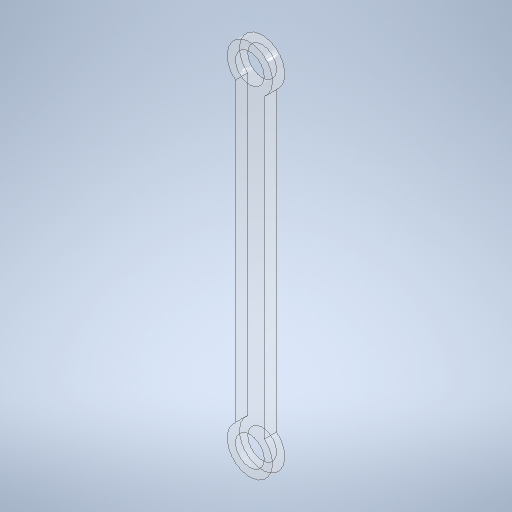
# Autodesk Inventor part: 4P.01.02.28-BC-v1-Final Aileron L3 80deg
Saved by Autodesk Inventor 2025.2 (Build 292293000, 293)
## iProperties
Created: 2025-01-30
Part Number: 4P.01.02.28-BC-v1-Final Aileron L3 80deg
Material: Acrylic, Clear
Document SubType Name: Modeling
Designer: Carriett 4
Density: 1.19 g/cm^3
Appearance: Transparent - Clear
Category: <PART CATAGORY>
Title: <TITLE>
Author: Carriett 4
Revision Number: 1
Autodesk Inventor part; units mm, degrees
ref_plane "YZ Plane" through (0, 0, 0) normal (1, 0, 0) x (0, 1, 0)
ref_plane "XZ Plane" through (0, 0, 0) normal (0, 1, 0) x (-1, 0, 0)
ref_plane "XY Plane" through (0, 0, 0) normal (0, 0, 1) x (1, 0, 0)
sketch "Sketch6" plane through (0, 0, 0) normal (0, 0, 1) x (1, 0, 0)
  arc A0 (9, 81.8659) -> (2, 81.8659) centre (5.5, 86.1086) ccw
  arc A1 (2, 9.7426) -> (9, 9.7426) centre (5.5, 5.5) ccw
  circle A2 centre (5.5, 5.5) radius 3.5
  circle A3 centre (5.5, 86.1086) radius 3.5
  line L0 (2, 81.8659) -> (2, 9.7426)
  line L1 (9, 9.7426) -> (9, 81.8659)
  point P0 (0, 0)
  dimension "d89" = 80.6086
  dimension "d90" = 7
  dimension "d91" = 7
  dimension "d92" = 5.5
  dimension "d93" = 7
  dimension "d94" = 5.5
  constraints: 4 centre point, 4 end point, 4 point on circle, 2 coincident, 2 tangent
  measures "d89" distance of A1.centre A0.centre
  measures "d90" distance between parallel lines of L1 L0
  measures "d91" diameter of A2
  measures "d92" radius of A1
  measures "d93" diameter of A3
  measures "d94" radius of A0
extrude "Extrusion3" add sketch "Sketch6" along normal blind 3
body "Solid2"
